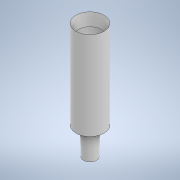
# Autodesk Inventor part: Pipet to Needle-tighter
Saved by Autodesk Inventor 2020 (Build 240168000, 168)
## iProperties
Created: 2020-08-22
Part Number: Pipet to Needle-tighter
Material: Generic
Document SubType Name: Modeling
Designer: pab2
Density: 1 g/cm^3
Appearance: Default
Author: pab2
Autodesk Inventor part; units mm, degrees
ref_plane "YZ Plane" through (0, 0, 0) normal (1, 0, 0) x (0, 1, 0)
ref_plane "XZ Plane" through (0, 0, 0) normal (0, 1, 0) x (-1, 0, 0)
ref_plane "XY Plane" through (0, 0, 0) normal (0, 0, 1) x (1, 0, 0)
sketch "Sketch1" plane through (0, 0, 0) normal (0, 0, 1) x (1, 0, 0)
  line L0 (0, 0) -> (2, 0)
  line L1 (2.225, 7.5) -> (2, 0)
  line L2 (2, 0) -> (1.5, 0)
  line L3 (1.5, 0) -> (1.5, 8.5)
  line L4 (2, 0) -> (1.5, 0)
  line L5 (0.1075, 35.8962) -> (4.3541, 35.8962) construction
  line L6 (3.5182, 32.4828) -> (4.3541, 35.8962)
  line L7 (3.5182, 32.4828) -> (28.4522, 32.4828) construction
  line L8 (1.5, 8.5) -> (3.5182, 10.5182)
  line L9 (1.5, 8.5) -> (4.3541, 8.5) construction
  line L10 (4.3541, 35.8962) -> (4.3541, 8.5)
  line L11 (2.225, 7.5) -> (4.3541, 8.5)
  line L12 (3.5182, 32.4828) -> (3.5182, 10.5182)
  line L13 (2, 0) -> (1.5, 0)
  line L14 (1.5, 0) -> (2, 0)
  line L15 (0, 0) -> (0, 42.8273)
  line L16 (0, 29.9682) -> (3.4162, 29.9682)
  dimension "d0" = 2
  dimension "d6" = 8.5
  dimension "d20" = 45
  constraints: 34 end point, 8 horizontal, 3 vertical, 2 perpendicular, 1 equal length, 1 point on line
  measures "d0" distance of L0.start L0.end
  measures "d6" distance of L2.end L3.end
  measures "d20" angle of L9 L8
revolve "Revolution1" add sketch "Sketch1" angle 360 about axis through (0, 0, 0) along (0, 1, 0)
body "Solid1"
